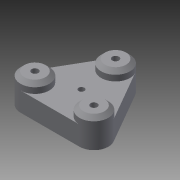
# Autodesk Inventor part: ShellFrame
Saved by Autodesk Inventor 2014 (Build 180170000, 170)
## iProperties
Created: 2016-01-26
Part Number: ShellFrame
Material: Generic
Document SubType Name: Modeling
Designer: Justin B
Density: 1 g/cm^3
Appearance: Default
Author: Justin B
Autodesk Inventor part; units mm, degrees
ref_plane "YZ Plane" through (0, 0, 0) normal (1, 0, 0) x (0, 1, 0)
ref_plane "XZ Plane" through (0, 0, 0) normal (0, 1, 0) x (-1, 0, 0)
ref_plane "XY Plane" through (0, 0, 0) normal (0, 0, 1) x (1, 0, 0)
sketch "Sketch1" plane through (0, 0, 0) normal (0, 0, 1) x (1, 0, 0)
  circle A0 centre (0, 0) radius 2 projected
  circle A1 centre (0, 17.3205) radius 2 projected
  circle A2 centre (-15, -8.6603) radius 2 projected
  circle A3 centre (15, -8.6603) radius 2 projected
  line L0 (-15, -16.1603) -> (15, -16.1603)
  line L1 (21.4952, -4.9103) -> (6.4952, 21.0705)
  line L2 (-6.4952, 21.0705) -> (-21.4952, -4.9103)
  arc A4 (6.4952, 21.0705) -> (-6.4952, 21.0705) centre (0, 17.3205) ccw
  arc A5 (15, -16.1603) -> (21.4952, -4.9103) centre (15, -8.6603) ccw
  arc A6 (-21.4952, -4.9103) -> (-15, -16.1603) centre (-15, -8.6603) ccw
  line L3 (15.512, -26.8675) -> (-15.512, -26.8675) projected
  line L4 (15.512, 26.8675) -> (31.0239, 0) projected
  line L5 (-31.0239, 0) -> (-15.512, 26.8675) projected
  line L6 (-31.0239, 0) -> (-15.512, -26.8675) projected
  line L7 (15.512, -26.8675) -> (31.0239, 0) projected
  line L8 (15.512, 26.8675) -> (-15.512, 26.8675) projected
  point P0 (0, 0)
  dimension "d3" = 7.5
  constraints: 7 point on circle, 6 end point, 6 tangent, 3 centre point, 3 coincident
  measures "d3" radius of A4
extrude "Extrusion1" add sketch "Sketch1" along normal blind 10 contours A0 | A1 | A2 | A3 | A6 L2 A4 L1 A5 L0
sketch "Sketch2" plane through (0, 0, 0) normal (0, 0, -1) x (-1, 0, 0)
  arc A0 (15, -16.1603) -> (21.4952, -4.9103) centre (15, -8.6603) ccw projected
  arc A1 (6.4952, 21.0705) -> (-6.4952, 21.0705) centre (0, 17.3205) ccw projected
  arc A2 (-21.4952, -4.9103) -> (-15, -16.1603) centre (-15, -8.6603) ccw projected
  point P0 (0, 0)
hole "Hole1" at (0, 17.3205, 0) at (15, -8.6603, 0) at (-15, -8.6603, 0) direction (0, 0, 1) diameter 4.5 depth 5.25
sketch "Sketch3" plane through (0, 0, 0) normal (0, 0, -1) x (-1, 0, 0)
  point P0 (0, 0)
hole "Hole2" at (0, 0, 0) direction (0, 0, 1) diameter 3 end through all
sketch "Sketch4" plane through (0, 0, 10) normal (0, 0, 1) x (1, 0, 0)
  arc A0 (15, -16.1603) -> (21.4952, -4.9103) centre (15, -8.6603) ccw projected
  arc A1 (6.4952, 21.0705) -> (-6.4952, 21.0705) centre (0, 17.3205) ccw projected
  arc A2 (-21.4952, -4.9103) -> (-15, -16.1603) centre (-15, -8.6603) ccw projected
  circle A3 centre (0, 17.3205) radius 7.5
  circle A4 centre (15, -8.6603) radius 7.5
  circle A5 centre (-15, -8.6603) radius 7.5
  constraints: 3 centre point, 3 coincident, 3 concentric
extrude "Extrusion2" add sketch "Sketch4" along normal blind 5
chamfer "Chamfer1" distance 2 angle 45 3 edges at (-22.5, -8.6603, 15) (-7.5, 17.3205, 15) (7.5, -8.6603, 15)
hole "Hole3" at (0, 17.3205, 15) direction (0, 0, -1) diameter 3.5 depth 6
hole "Hole4" at (15, -8.6603, 15) direction (0, 0, -1) diameter 3.5 depth 6
hole "Hole5" at (-15, -8.6603, 15) direction (0, 0, -1) diameter 3.5 depth 6
body "Solid1"
